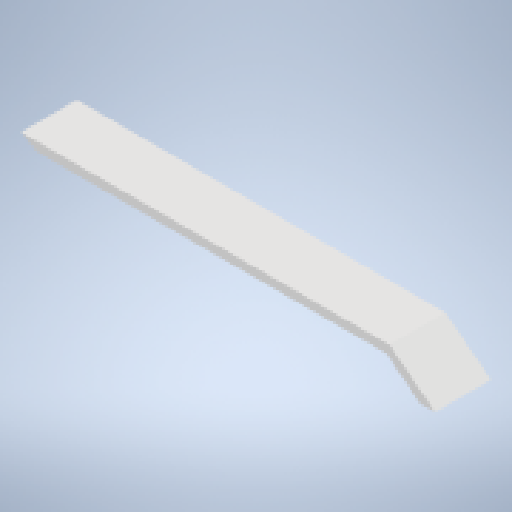
# Autodesk Inventor part: handle
Saved by Autodesk Inventor 2025 (Build 290162000, 162)
## iProperties
Created: 2026-09-07
Part Number: handle
Material: Типовые
Document SubType Name: Modeling
Designer: Leva
Density: 1 g/cm^3
Appearance: По умолчанию
Author: Leva
Autodesk Inventor part; units mm, degrees
ref_plane "YZ Plane" through (0, 0, 0) normal (1, 0, 0) x (0, 1, 0)
ref_plane "XZ Plane" through (0, 0, 0) normal (0, 1, 0) x (-1, 0, 0)
ref_plane "XY Plane" through (0, 0, 0) normal (0, 0, 1) x (1, 0, 0)
sketch "Эскиз1" plane through (0, 0, 0) normal (0, 0, 1) x (1, 0, 0)
  line L0 (176.9, 11.5) -> (160.5, 11.5) projected
  line L1 (19.5, 13.5) -> (19.5, 3.5) projected
  line L2 (19.5, 3.5) -> (127.2, 3.5) projected
  line L3 (127.2, 3.5) -> (127.2, -1.5) projected
  line L4 (127.2, -1.5) -> (2.5, -1.5) projected
  line L5 (2.5, -1.5) -> (2.5, 18.5) projected
  line L6 (2.5, 18.5) -> (36.5, 18.5) projected
  line L7 (36.5, 18.5) -> (36.5, 13.5) projected
  line L8 (36.5, 13.5) -> (19.5, 13.5) projected
  line L9 (131.9067, -6.5) -> (131.9067, 11.5) projected
  line L10 (131.9067, 11.5) -> (59.18, 11.5) projected
  line L11 (59.18, 11.5) -> (51.5, 15.5635) projected
  line L12 (36.5, 23.5) -> (-2.5, 23.5) projected
  line L13 (-2.5, 23.5) -> (-2.5, 12.5) projected
  line L14 (-2.5, 12.5) -> (0.5, 12.5) projected
  line L15 (0.5, 12.5) -> (0.5, 9.5) projected
  line L16 (0.5, 9.5) -> (-2.5, 9.5) projected
  line L17 (-2.5, 9.5) -> (-2.5, -3.5) projected
  line L18 (5.5, -6.5) -> (131.9067, -6.5) projected
  circle A0 centre (129.7, 9) radius 1.25 projected
  line L19 (36.5, 23.5) -> (161.5, 23.5)
  line L20 (161.5, 23.5) -> (176.9, 11.5)
  line L21 (176.9, 11.5) -> (171.9, 11.5)
  line L22 (171.9, 11.5) -> (160.35, 20.5)
  line L23 (36.5, 23.5) -> (36.5, 20.5)
  line L24 (36.5, 20.5) -> (160.35, 20.5)
  line L25 (42.17, 20.5) -> (36.5, 23.5) projected
  line L26 (51.5, 20.5) -> (51.5, 15.5635) projected
  line L27 (42.17, 20.5) -> (51.5, 20.5) projected
  line L28 (5.5, -6.5) -> (5.5, -3.5) projected
  line L29 (-2.5, -3.5) -> (5.5, -3.5) projected
  point P0 (0, 0)
  point P1 (42.17, 20.5)
  dimension "d0" = 125
  dimension "d1" = 5
  dimension "d2" = 3
  constraints: 12 end point, 3 parallel, 1 point on line, 1 vertical
  measures "d0" distance of L12.start L19.end
  measures "d1" distance of L0.start L21.end
  measures "d2" distance of L12.start L23.end
extrude "Выдавливание1" add sketch "Эскиз1" against normal blind 19 contours L0 L22 L24 L25 L19 L20 | L25 L24 L23
sketch "Эскиз2" plane through (36.5, 23.5, 0) normal (0, 1, 0) x (1, 0, 0)
  line L0 (125, 0) -> (0, 0) projected
  line L1 (0, 19) -> (125, 19) projected
  line L2 (0, 0) -> (10.335, 0) construction
  line L3 (10.335, 0) -> (10.335, 19) construction
  line L4 (10.335, 19) -> (0, 19) construction
  line L5 (0, 19) -> (0, 0) construction
  circle A0 centre (10.335, 9.5) radius 1.25
  point P0 (-36.5, 0)
  dimension "d5" = 10.335
  dimension "d6" = 2.5
  constraints: 8 end point, 2 parallel, 1 centre point, 1 horizontal, 1 midpoint, 1 perpendicular, 1 point on line
  measures "d5" distance of L4.end L3.end
  measures "d6" diameter of A0
extrude "Выдавливание2" cut sketch "Эскиз2" against normal blind 3
sketch "Эскиз3" plane through (171.9, 11.5, 0) normal (0, -1, 0) x (1, 0, 0)
  line L0 (5, 0) -> (-10.4, 0) projected
  line L1 (5, 0) -> (-1, 0)
  line L2 (-1, 0) -> (-1, 5)
  line L3 (-1, 5) -> (5, 5)
  line L4 (5, 5) -> (5, 0)
  line L5 (-1, 2.5) -> (5, 2.5) construction
  line L6 (2, 5) -> (2, 0) construction
  circle A0 centre (2, 2.5) radius 1.25
  line L7 (5, 0) -> (5, -19) construction
  line L8 (5, 0) -> (5, -19) construction
  line L9 (5, 0) -> (5, -19) construction
  line L10 (5, -9.5) -> (-10.4, -9.5) construction
  line L11 (-10.4, 0) -> (-10.4, -19) construction
  line L12 (5, -19) -> (-1, -19)
  line L13 (-1, -19) -> (-1, -24)
  line L14 (-1, -24) -> (5, -24)
  line L15 (5, -24) -> (5, -19)
  line L16 (-1, -21.5) -> (5, -21.5) construction
  line L17 (2, -24) -> (2, -19) construction
  circle A1 centre (2, -21.5) radius 1.25
  point P0 (-171.9, 0)
  point P1 (-1, 0)
  dimension "d9" = 6
  dimension "d10" = 5
  dimension "d11" = 2.5
  constraints: 30 end point, 8 symmetric about line, 7 midpoint, 4 equal length, 2 centre point, 1 horizontal, 1 perpendicular, 1 other
  measures "d9" distance of L2.end L3.end
  measures "d10" distance of L1.end L2.end
  measures "d11" diameter of A0
extrude "Выдавливание3" add sketch "Эскиз3" against normal blind 2
chamfer "Фаска1" distance 1.5775 angle 45 2 edges at (175.6167, 12.5, -19) (175.6167, 12.5, 0)
fillet "Сопряжение1" radius 1 4 edges at (170.9, 12.5, 5) (176.9, 12.5, 5) (176.9, 12.5, -24) (170.9, 12.5, -24)
chamfer "Фаска2" distance 5.7 distance2 3 1 edges at (36.5, 20.5, -9.5) measured on face at (122.9283, 20.5, -9.5)
chamfer "Фаска3" distance 0.614 angle 45 2 edges at (171.4, 11.8896, 0) (171.4, 11.8896, -19)
